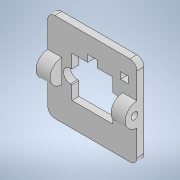
# Autodesk Inventor part: Крепление камеры
Saved by Autodesk Inventor 2020 (Build 240168000, 168)
## iProperties
Created: 2021-04-12
Part Number: Крепление камеры
Material: Типовые
Document SubType Name: Modeling
Designer: Антон
Density: 1 g/cm^3
Appearance: По умолчанию
Author: Антон
Autodesk Inventor part; units mm, degrees
ref_plane "YZ Plane" through (0, 0, 0) normal (1, 0, 0) x (0, 1, 0)
ref_plane "XZ Plane" through (0, 0, 0) normal (0, 1, 0) x (-1, 0, 0)
sketch "Эскиз2" plane through (0, 0, 0) normal (0, 0, 1) x (1, 0, 0)
  line L0 (0, 0) -> (38, 0)
  line L1 (38, 0) -> (38, 38)
  line L2 (38, 38) -> (0, 38)
  line L3 (0, 38) -> (0, 0)
  line L4 (0, 38) -> (10.3, 38)
  line L5 (10.3, 38) -> (10.3, 27.7)
  line L6 (10.3, 27.7) -> (27.7, 27.7)
  line L7 (27.7, 27.7) -> (27.7, 10.3)
  line L8 (27.7, 10.3) -> (10.3, 10.3)
  line L9 (10.3, 10.3) -> (10.3, 27.7)
  line L10 (10.3, 27.7) -> (10.3, 21.9)
  line L11 (10.3, 21.9) -> (6.7, 21.9)
  line L12 (6.7, 21.9) -> (6.7, 16.1)
  line L13 (6.7, 16.1) -> (10.3, 16.1)
  line L14 (10.3, 16.1) -> (10.3, 21.9)
  line L15 (6.7, 19) -> (7.7, 19)
  circle A0 centre (7.7, 19) radius 0.5
  line L16 (19, 27.7) -> (19, 10.3)
  line L17 (27.7, 21.9) -> (31.3, 21.9)
  line L18 (31.3, 21.9) -> (31.3, 16.1)
  line L19 (31.3, 16.1) -> (27.7, 16.1)
  line L20 (27.7, 16.1) -> (27.7, 21.9)
  line L21 (31.3, 19) -> (30.3, 19)
  circle A1 centre (30.3, 19) radius 0.5
  line L22 (19, 27.7) -> (19, 29.2)
  line L23 (21, 30.7) -> (21, 27.7)
  line L24 (21, 27.7) -> (17, 27.7)
  line L25 (17, 27.7) -> (17, 30.7)
  line L26 (17, 30.7) -> (21, 30.7)
  line L27 (21, 30.7) -> (17, 27.7) construction
  line L28 (21, 27.7) -> (17, 30.7) construction
  point P0 (27.7, 21.9)
  point P1 (27.7, 16.1)
  point P2 (10.3, 16.1)
  dimension "d11" = 38
  dimension "d12" = 38
  dimension "d55" = 10.3
  dimension "d56" = 10.3
  dimension "d57" = 17.4
  dimension "d58" = 17.4
  dimension "d59" = 5.8
  dimension "d60" = 3.6
  dimension "d61" = 5.8
  dimension "d62" = 1
  dimension "d63" = 1
  dimension "d85" = 1.5
  dimension "d86" = 4
  constraints: 58 end point, 8 parallel, 7 midpoint, 7 symmetric about line, 6 perpendicular, 4 horizontal, 2 centre point, 2 coincident, 2 point on line, 1 vertical, 1 other
  measures "d11" distance of L2.end L1.end
  measures "d12" distance of L1.end L0.end
  measures "d55" distance of L2.end L4.end
  measures "d56" distance of L4.end L5.end
  measures "d57" distance of L7.end L8.end
  measures "d58" distance of L6.end L7.end
  measures "d59" distance of L5.end L10.end
  measures "d60" distance of L13.end L12.end
  measures "d61" distance of L12.end L11.end
  measures "d62" distance of L15.start L15.end
  measures "d63" diameter of A0
  measures "d85" distance of L16.start L22.end
  measures "d86" distance of L23.end L24.end
extrude "Выдавливание1" add sketch "Эскиз2" along normal blind 3 contours L3 L2 L1 L0
sketch "Эскиз4" plane through (35, 35, 0) normal (0, 0, -1) x (-1, 0, 0)
  circle A0 centre (0, 0) radius 3 projected
  arc A1 (32, 3) -> (35, 0) centre (32, 0) ccw projected
  circle A2 centre (0, -32) radius 3 projected
  circle A3 centre (32, -32) radius 3 projected
  point P0 (35, -35)
  constraints: 4 coincident
hole "Отверстие1" at (35, 35, 0) at (3, 35, 0) at (35, 3, 0) at (3, 3, 0) direction (0, 0, 1) diameter 2.95 depth 2
fillet "Сопряжение1" radius 2.9 4 edges at (6.7, 21.9, 1.5) (6.7, 16.1, 1.5) (31.3, 16.1, 1.5) (31.3, 21.9, 1.5)
sketch "Эскиз6" plane through (0, 0, 3) normal (0, 0, 1) x (1, 0, 0)
  line L0 (38, 38) -> (0, 38) projected
  line L1 (38, 38) -> (38, 31.3)
  line L2 (38, 0) -> (38, 38) projected
  line L3 (38, 31.3) -> (34.3, 31.3)
  line L4 (34.3, 31.3) -> (31, 31.3)
  line L5 (31, 31.3) -> (31, 28.5)
  line L6 (31, 28.5) -> (34.3, 28.5)
  line L7 (34.3, 28.5) -> (34.3, 31.3)
  point P0 (0, 0)
  point P1 (35, 38)
  point P2 (38, 3)
  point P3 (38, 35)
  dimension "d65" = 6.7
  dimension "d66" = 3.7
  dimension "d67" = 3.3
  dimension "d68" = 2.8
  constraints: 12 end point, 2 horizontal, 2 parallel, 1 perpendicular, 1 point on line
  measures "d65" distance of L0.start L1.end
  measures "d66" distance of L1.end L3.end
  measures "d67" distance of L6.end L5.end
  measures "d68" distance of L5.end L4.end
extrude "Выдавливание4" cut sketch "Эскиз6" against normal through all
sketch "Эскиз7" plane through (0, 0, 3) normal (0, 0, 1) x (1, 0, 0)
  line L0 (0, 38) -> (0, 0) projected
  line L1 (0, 19) -> (3, 19)
  line L2 (6, 14) -> (6, 24)
  line L3 (6, 24) -> (0, 24)
  line L4 (0, 24) -> (0, 14)
  line L5 (0, 14) -> (6, 14)
  line L6 (6, 14) -> (0, 24) construction
  line L7 (6, 24) -> (0, 14) construction
  dimension "d83" = 3
  dimension "d84" = 10
  constraints: 14 end point, 3 midpoint, 2 parallel, 1 collinear, 1 horizontal, 1 perpendicular, 1 vertical
  measures "d83" distance of L1.start L1.end
  measures "d84" distance of L2.start L2.end
extrude "Выдавливание5" add sketch "Эскиз7" along normal blind 5
fillet "Сопряжение2" radius 5 2 edges at (3, 14, 8) (3, 24, 8)
sketch "Эскиз8" plane through (0, 0, 0) normal (-1, 0, 0) x (0, 0, 1)
  line L0 (0, 38) -> (0, 0) projected
  line L1 (0, 19) -> (8, 19)
  arc A0 (3, 14) -> (3, 24) centre (3, 19) ccw projected
  point P0 (4, 19)
  constraints: 2 end point, 2 midpoint, 1 perpendicular, 1 point on circle
hole "Отверстие2" at (0, 19, 4) direction (1, 0, 0) diameter 2.95 depth 5
ref_plane "РабПлоскость1" through (19, 0, 0) normal (-1, 0, 0) x (0, 0, 1)
fillet "Сопряжение3" radius 3 4 edges at (38, 38, 1.5) (0, 38, 1.5) (0, 0, 1.5) (38, 0, 1.5)
sketch "Эскиз9" plane through (0, 19, 3) normal (-1, 0, 0) x (0, 0, 1)
  line L0 (-3, 16) -> (-3, -16) projected
  circle A0 centre (1, 0) radius 1.475 projected
  line L1 (2.5011, 2.6) -> (4.0022, 0)
  line L2 (4.0022, 0) -> (2.5011, -2.6)
  line L3 (2.5011, -2.6) -> (-0.5011, -2.6)
  line L4 (-0.5011, -2.6) -> (-2.0022, 0)
  line L5 (-2.0022, 0) -> (-0.5011, 2.6)
  line L6 (-0.5011, 2.6) -> (2.5011, 2.6)
  line L7 (-0.5011, 2.6) -> (-3, 2.6)
  line L8 (-3, 2.6) -> (-3, -2.6)
  line L9 (-3, -2.6) -> (-0.5011, -2.6)
  line L10 (-0.5011, -2.6) -> (-0.5011, 2.6)
  point P0 (-3, -19)
  point P1 (-3, 2.6)
  point P2 (-3, -2.6)
  point P3 (-0.5011, -2.6)
  dimension "d91" = 5.2
  constraints: 20 end point, 2 collinear, 2 parallel, 2 perpendicular, 1 coincident, 1 horizontal, 13 other
  measures "d91" distance between parallel lines of L3 L6
extrude "Выдавливание6" cut sketch "Эскиз9" along normal blind 3 from surface at -5 contours L7 L5 L4 L9 L0 | L10 L4 L5 | L6 L1 L2 L3 L10 | A0
mirror "Зеркальное отражение2" about plane through (19, 0, 0) normal (-1, 0, 0) of "Сопряжение2", "Отверстие2", "Выдавливание6", "Выдавливание5"
equation "\"d55\" = -0.5 * d57 + 0.5 * d11"
equation "\"d56\" = -0.5 * d58 + 0.5 * d12"
equation "\"d59\" = -0.5 * d61 + 0.5 * d58"
